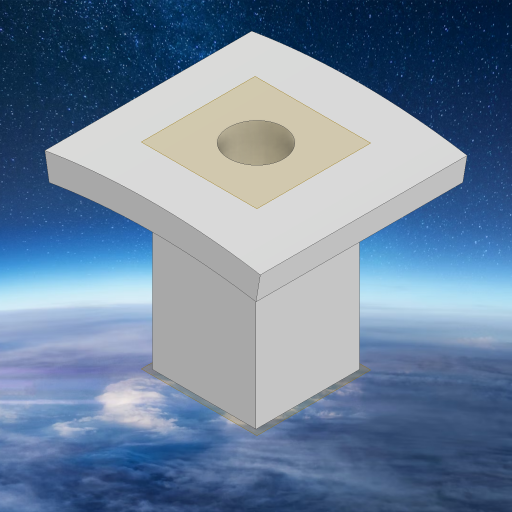
# Autodesk Inventor part: shiftt_fixed_plate
Saved by Autodesk Inventor 2023 (Build 270158000, 158)
## iProperties
Created: 2023-10-23
Part Number: shiftt_fixed_plate
Material: 一般
Document SubType Name: Modeling
Designer: 310611102
Density: 1 g/cm^3
Appearance: 預設
Author: 310611102
Autodesk Inventor part; units mm, degrees
ref_plane "YZ Plane" through (0, 0, 0) normal (1, 0, 0) x (0, 1, 0)
ref_plane "XY Plane" through (0, 0, 0) normal (0, 0, 1) x (1, 0, 0)
sketch "Sketch1" plane through (0, 0, 0) normal (0, 0, 1) x (1, 0, 0)
  arc A0 (20.833333, 123.251662) -> (-20.833333, 123.251662) centre (0, 0) ccw
  arc A1 (20, 118.321596) -> (-20, 118.321596) centre (0, 0) ccw
  line L0 (-20, 118.321596) -> (-20.833333, 123.251662)
  line L1 (0, 0) -> (0, 133.48158) construction
  line L2 (20, 118.321596) -> (20.833333, 123.251662)
  dimension "d0" = 250
  dimension "d1" = 5
  dimension "d2" = 40
  constraints: 6 end point, 4 point on circle, 2 centre point, 2 symmetric about line, 1 coincident, 1 line through centre, 1 vertical
  measures "d0" diameter of A0
  measures "d1" radial gap between concentric circles of A0 A1
  measures "d2" distance of L2.start L0.start
extrude "Extrusion1" add sketch "Sketch1" along normal mid plane 40
ref_plane "Work Plane3" through (0, 87, 0) normal (0, 1, 0) x (-1, 0, 0)
ref_plane "Work Plane2" through (0, 125, 0) normal (0, 1, 0) x (-1, 0, 0)
sketch "Sketch3" plane through (0, 87, 0) normal (0, 1, 0) x (-1, 0, 0)
  line L0 (10, -10) -> (-10, -10)
  line L1 (-10, -10) -> (-10, 10)
  line L2 (-10, 10) -> (10, 10)
  line L3 (10, 10) -> (10, -10)
  line L4 (10, -10) -> (-10, 10) construction
  line L5 (-10, -10) -> (10, 10) construction
  point P0 (0, 0)
  dimension "d6" = 20
  dimension "d7" = 20
  constraints: 12 end point, 2 midpoint, 2 parallel, 1 horizontal, 1 perpendicular
  measures "d6" distance of L0.start L0.end
  measures "d7" distance of L0.end L1.end
extrude "Extrusion2" add sketch "Sketch3" along normal up to next
sketch "Sketch4" plane through (0, 125, 0) normal (0, 1, 0) x (-1, 0, 0)
  circle A0 centre (0, 0) radius 5.3
  dimension "d10" = 10.6
  constraints: 1 centre point, 1 coincident
  measures "d10" diameter of A0
extrude "Extrusion3" cut sketch "Sketch4" against normal blind 34
body "Solid1"
